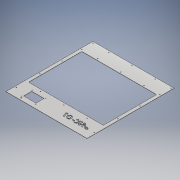
# Autodesk Inventor part: Front Cladding
Saved by Autodesk Inventor 2019 (Build 230136000, 136)
## iProperties
Created: 2018-10-13
Part Number: Front Cladding
Material: Aluminium 1050
Document SubType Name: Sheet Metal
Designer: Ax
Density: 2.7 g/cm^3
Sheet Metal Rule: Default_mm
Appearance: Anodized - Black
Mass: 471.716 g
Surface Area: 2405.62 cm^2
Volume: 174.71 cm^3
Flat Pattern Width: 51.3 cm
Flat Pattern Length: 55 cm
Flat Pattern Area: 2821.5 cm^2
Sheet Metal Width: 513.000 mm
Sheet Metal Length: 550.000 mm
Sheet Metal Area: 282150.000 mm^2
Author: Ax
Autodesk Inventor part; units mm, degrees
ref_plane "YZ Plane" through (0, 0, 0) normal (1, 0, 0) x (0, 1, 0)
ref_plane "XZ Plane" through (0, 0, 0) normal (0, 1, 0) x (-1, 0, 0)
ref_plane "XY Plane" through (0, 0, 0) normal (0, 0, 1) x (1, 0, 0)
sketch "Sketch6" plane through (0, 0, 0) normal (0, 0, -1) x (-1, 0, 0)
  line L0 (-182.0134, -208.3085) -> (-165.3558, -208.3085)
  line L1 (-165.3558, -208.3085) -> (-165.3558, -210.3085)
  line L2 (-165.3558, -210.3085) -> (-182.0134, -210.3085)
  line L3 (-182.0134, -210.3085) -> (-182.0134, -208.3085)
  line L4 (-85.6501, -195.172) -> (-83.6501, -195.172)
  line L5 (-83.6501, -195.172) -> (-83.6501, -232.9934)
  line L6 (-83.6501, -232.9934) -> (-85.6501, -232.9934)
  line L7 (-85.6501, -232.9934) -> (-85.6501, -195.172)
  line L8 (-204.8344, -216.2286) -> (-188.1555, -229.1813)
  line L9 (-188.1555, -229.1813) -> (-186.9288, -227.6017)
  line L10 (-186.9288, -227.6017) -> (-203.6076, -214.649)
  line L11 (-203.6076, -214.649) -> (-204.8344, -216.2286)
  point P0 (0, 0)
  dimension "d49" = 2
  dimension "d51" = 2
  dimension "d52" = 37.8214
  measures "d49" distance of L0.end L1.end
  measures "d51" distance of L4.start L4.end
  measures "d52" distance of L6.end L4.start
sketch "Sketch1" plane through (0, 0, 0) normal (0, 0, 1) x (1, 0, 0)
  line L0 (-256.5, -275) -> (256.5, -275)
  line L1 (256.5, -275) -> (256.5, 275)
  line L2 (256.5, 275) -> (-256.5, 275)
  line L3 (-256.5, 275) -> (-256.5, -275)
  line L4 (-256.5, -275) -> (256.5, 275) construction
  line L5 (256.5, -275) -> (-256.5, 275) construction
  line L6 (-256.5, 265) -> (256.5, 265) construction
  line L7 (-246.5, 275) -> (-246.5, -275) construction
  line L8 (246.5, 275) -> (246.5, -275) construction
  line L9 (-256.5, -165) -> (256.5, -165) construction
  line L10 (-256.5, 195) -> (256.5, 195) construction
  circle A0 centre (-246.5, 265) radius 2.1
  circle A1 centre (-146.5, 265) radius 2.1
  circle A2 centre (146.5, 265) radius 2.1
  circle A3 centre (246.5, 265) radius 2.1
  circle A4 centre (146.5, 195) radius 2.1
  circle A5 centre (246.5, 195) radius 2.1
  circle A6 centre (-246.5, 195) radius 2.1
  circle A7 centre (-146.5, 195) radius 2.1
  line L11 (-146.5, 275) -> (-146.5, -275) construction
  line L12 (0, 0) -> (0, -275) construction
  line L13 (146.5, 275) -> (146.5, -275) construction
  circle A8 centre (-246.5, 70) radius 2.1
  circle A9 centre (146.5, -165) radius 2.1
  circle A10 centre (-146.5, -165) radius 2.1
  circle A11 centre (-246.5, -70) radius 2.1
  circle A12 centre (-246.5, -220) radius 2.1
  circle A13 centre (246.5, -220) radius 2.1
  circle A14 centre (246.5, -70) radius 2.1
  circle A15 centre (246.5, 70) radius 2.1
  line L14 (-246.5, 70) -> (246.5, 70) construction
  line L15 (-246.5, -70) -> (246.5, -70) construction
  line L16 (-246.5, 0) -> (246.5, 0) construction
  line L17 (-246.5, -220) -> (246.5, -220) construction
  line L18 (0, 275) -> (0, 0) construction
  circle A16 centre (0, 265) radius 2.1
  circle A17 centre (0, 195) radius 2.1
  circle A18 centre (0, -165) radius 2.1
  line L19 (-236.5, -152) -> (236.5, -152)
  line L20 (236.5, -152) -> (236.5, 185)
  line L21 (236.5, 185) -> (-236.5, 185)
  line L22 (-236.5, 185) -> (-236.5, -152)
  dimension "d0" = 513
  dimension "d1" = 550
  dimension "d2" = 10
  dimension "d3" = 10
  dimension "d4" = 10
  dimension "d5" = 110
  dimension "d6" = 80
  dimension "d7" = 110
  dimension "d8" = 110
  dimension "d9" = 70
  dimension "d10" = 55
  dimension "d11" = 4.2
  dimension "d14" = 10
  dimension "d15" = 10
  dimension "d17" = 13
  dimension "d18" = 10
  measures "d0" distance of L1.end L2.end
  measures "d1" distance of L0.end L1.end
  measures "d2" distance of L2.end L6.start
  measures "d3" distance of L0.start L7.end
  measures "d4" distance of L0.end L8.end
  measures "d5" distance of L0.end L9.end
  measures "d6" distance of L10.end L1.end
  measures "d7" distance of L0.start L11.end
  measures "d8" distance of L13.end L0.end
  measures "d9" vertical distance of L12.start L14.start
  measures "d10" vertical distance of L0.end L17.end
  measures "d11" diameter of A7
  measures "d14" distance between parallel lines of L10 L21
  measures "d15" distance between parallel lines of L8 L20
  measures "d17" distance from line of L9 L19.end
  measures "d18" distance between parallel lines of L7 L22
extrude "Plate4" add sketch "Sketch1" along normal blind 1.5
fillet "Fillet1" radius 5 4 edges at (-236.5, 185, 0.75) (236.5, 185, 0.75) (236.5, -152, 0.75) (-236.5, -152, 0.75)
sketch "Sketch2" plane through (0, 0, 1.5) normal (0, 0, 1) x (1, 0, 0)
  line L0 (-176.5, -192) -> (-98.05, -192)
  line L1 (-98.05, -192) -> (-98.05, -243)
  line L2 (-98.05, -243) -> (-176.5, -243)
  line L3 (-176.5, -243) -> (-176.5, -192)
  line L4 (256.5, 275) -> (256.5, -275) projected
  line L5 (231.5, -152) -> (-231.5, -152) projected
  line L6 (-256.5, -275) -> (-256.5, 275) projected
  point P0 (0, 0)
  dimension "d22" = 78.45
  dimension "d23" = 51
  dimension "d25" = 40
  dimension "d28" = 80
  constraints: 8 end point, 2 parallel, 1 horizontal, 1 perpendicular
  measures "d22" distance of L0.start L0.end
  measures "d23" distance of L0.end L1.end
  measures "d25" distance between parallel lines of L0 L5
  measures "d28" distance between parallel lines of L3 L6
extrude "Cut1" cut sketch "Sketch2" against normal blind 1.5
sketch "Sketch3" plane through (0, 0, 0) normal (0, 0, -1) x (-1, 0, 0)
  circle A0 centre (173.45, -261.3) radius 3.25
  line L0 (176.5, -243) -> (98.05, -243) projected
  point P0 (0, 0)
  dimension "d29" = 6.5
  dimension "d30" = 18.3
  dimension "d31" = 3.05
  constraints: 1 centre point
  measures "d29" diameter of A0
  measures "d30" distance from line of A0.centre L0
  measures "d31" horizontal distance of L0.start A0.centre
extrude "Cut2" cut sketch "Sketch3" against normal blind 1.5
sketch "Sketch4" plane through (0, 0, 0) normal (0, 0, -1) x (-1, 0, 0)
  line L0 (93.3, -250) -> (181.25, -250) construction
  line L1 (181.25, -250) -> (181.25, -185) construction
  line L2 (181.25, -185) -> (93.3, -185) construction
  line L3 (93.3, -185) -> (93.3, -250) construction
  line L4 (93.3, -250) -> (181.25, -185) construction
  line L5 (181.25, -250) -> (93.3, -185) construction
  line L6 (98.05, -243) -> (98.05, -192) construction
  line L7 (98.05, -217.5) -> (176.5, -217.5) construction
  line L8 (176.5, -192) -> (176.5, -243) construction
  circle A0 centre (181.25, -185) radius 1.7
  circle A1 centre (181.25, -250) radius 1.7
  circle A2 centre (93.3, -250) radius 1.7
  circle A3 centre (93.3, -185) radius 1.7
  point P0 (0, 0)
  point P1 (137.275, -217.5)
  point P2 (137.275, -217.5)
  dimension "d34" = 87.95
  dimension "d35" = 65
  dimension "d36" = 3.4
  constraints: 14 end point, 6 midpoint, 4 centre point, 4 coincident, 3 equal radius, 2 parallel, 2 perpendicular, 1 horizontal
  measures "d34" distance of L0.start L0.end
  measures "d35" distance of L2.end L0.start
  measures "d36" diameter of A0
hole "Hole1" at (-181.25, -250, 0) at (-181.25, -185, 0) at (-93.3, -185, 0) at (-93.3, -250, 0) direction (0, 0, 1) diameter 3.4 end through all
sketch "Sketch5" plane through (0, 0, 0) normal (0, 0, -1) x (-1, 0, 0)
  line L0 (-179.5318, -196.7353) -> (-76.9682, -196.7353) construction
  line L1 (-76.9682, -196.7353) -> (-76.9682, -230.2647) construction
  line L2 (-76.9682, -230.2647) -> (-179.5318, -230.2647) construction
  line L3 (-179.5318, -230.2647) -> (-179.5318, -196.7353) construction
  line L4 (-128.25, -196.7353) -> (-128.25, -230.2647) construction
  line L5 (231.5, -152) -> (-231.5, -152) projected
  line L6 (-256.5, -275) -> (-256.5, 275) projected
  spline S0 degree 2 poles (-150.7053, -213.6532) (-151.7777, -217.0234) (-155.8628, -217.0234) knots 0 0 0 1 1 1
  line L7 (-155.8628, -217.0234) -> (-168.3989, -217.0234)
  line L8 (-168.3989, -217.0234) -> (-172.3564, -228.0021)
  line L9 (-172.3564, -228.0021) -> (-179.9138, -228.0021)
  line L10 (-179.9138, -228.0021) -> (-175.9564, -217.0234)
  line L11 (-175.9564, -217.0234) -> (-182.4415, -217.0234)
  spline S1 degree 2 poles (-182.4415, -217.0234) (-193.0628, -229.866) (-203.2245, -229.866) knots 0 0 0 1 1 1
  spline S2 degree 2 poles (-203.2245, -229.866) (-206.1862, -229.866) (-208.2032, -228.7681) knots 0 0 0 1 1 1
  spline S3 degree 2 poles (-208.2032, -228.7681) (-210.7564, -227.3638) (-210.7564, -224.683) knots 0 0 0 1 1 1
  spline S4 degree 2 poles (-210.7564, -224.683) (-210.7564, -222.3596) (-208.867, -220.1638) knots 0 0 0 1 1 1
  spline S5 degree 2 poles (-208.867, -220.1638) (-205.8032, -216.6404) (-199.5989, -214.9553) knots 0 0 0 1 1 1
  spline S6 degree 2 poles (-199.5989, -214.9553) (-194.7479, -213.6532) (-188.8755, -213.6532) knots 0 0 0 1 1 1
  line L12 (-188.8755, -213.6532) -> (-184.7904, -213.6532)
  line L13 (-184.7904, -213.6532) -> (-172.05, -198.3085)
  line L14 (-172.05, -198.3085) -> (-161.8117, -198.3085)
  line L15 (-161.8117, -198.3085) -> (-167.25, -213.6532)
  line L16 (-167.25, -213.6532) -> (-150.7053, -213.6532)
  spline S7 degree 2 poles (-187.6245, -217.0234) (-195.5394, -217.0234) (-198.7309, -219.2957) knots 0 0 0 1 1 1
  spline S8 degree 2 poles (-198.7309, -219.2957) (-201.3606, -221.2106) (-201.3606, -223.3553) knots 0 0 0 1 1 1
  spline S9 degree 2 poles (-201.3606, -223.3553) (-201.3606, -225.1681) (-199.4713, -225.1681) knots 0 0 0 1 1 1
  spline S10 degree 2 poles (-199.4713, -225.1681) (-196.8415, -225.1681) (-192.9351, -222.2064) knots 0 0 0 1 1 1
  spline S11 degree 2 poles (-192.9351, -222.2064) (-189.4883, -219.6532) (-187.6245, -217.0234) knots 0 0 0 1 1 1
  line L17 (-170.3904, -201.8064) -> (-179.633, -213.6532)
  line L18 (-179.633, -213.6532) -> (-174.9351, -213.6532)
  line L19 (-174.9351, -213.6532) -> (-170.3904, -201.8064)
  spline S12 degree 2 poles (-119.1989, -202.1894) (-119.1989, -204.3851) (-120.9351, -205.8404) knots 0 0 0 1 1 1
  spline S13 degree 2 poles (-120.9351, -205.8404) (-122.5692, -207.2447) (-124.7649, -207.2447) knots 0 0 0 1 1 1
  spline S14 degree 2 poles (-124.7649, -207.2447) (-126.2457, -207.2447) (-129.1819, -205.7128) (-129.9734, -204.4872) knots 0 0 0 1 2 2 2
  line L20 (-129.9734, -204.4872) -> (-137.0968, -211.9681)
  line L21 (-137.0968, -211.9681) -> (-133.7777, -224.6319)
  line L22 (-133.7777, -224.6319) -> (-122.7479, -224.6319)
  spline S15 degree 2 poles (-122.7479, -224.6319) (-123.0287, -226.2915) (-124.7649, -227.2106) knots 0 0 0 1 1 1
  spline S16 degree 2 poles (-124.7649, -227.2106) (-126.2202, -228.0021) (-128.0585, -228.0021) knots 0 0 0 1 1 1
  line L23 (-128.0585, -228.0021) -> (-136.3564, -228.0021)
  spline S17 degree 2 poles (-136.3564, -228.0021) (-138.4245, -228.0021) (-139.9053, -226.7511) knots 0 0 0 1 1 1
  spline S18 degree 2 poles (-139.9053, -226.7511) (-141.3096, -225.5511) (-141.8968, -223.5596) knots 0 0 0 1 1 1
  line L24 (-141.8968, -223.5596) -> (-143.3266, -218.683)
  line L25 (-143.3266, -218.683) -> (-150.067, -225.7043)
  spline S19 degree 2 poles (-150.067, -225.7043) (-152.7989, -228.5638) (-155.9394, -228.5638) knots 0 0 0 1 1 1
  spline S20 degree 2 poles (-155.9394, -228.5638) (-158.1606, -228.5638) (-159.8202, -227.1596) knots 0 0 0 1 1 1
  spline S21 degree 2 poles (-159.8202, -227.1596) (-161.5564, -225.7043) (-161.5564, -223.483) knots 0 0 0 1 1 1
  spline S22 degree 2 poles (-161.5564, -223.483) (-161.5564, -221.3894) (-158.2628, -218.4277) (-155.9394, -218.4277) knots 0 0 0 1 2 2 2
  spline S23 degree 2 poles (-155.9394, -218.4277) (-152.4415, -218.4277) (-150.884, -221.3383) knots 0 0 0 1 1 1
  line L26 (-150.884, -221.3383) -> (-144.45, -214.5979)
  line L27 (-144.45, -214.5979) -> (-147.0287, -203.6191)
  line L28 (-147.0287, -203.6191) -> (-157.5223, -203.6191)
  line L29 (-157.5223, -203.6191) -> (-154.3309, -198.3085)
  line L30 (-154.3309, -198.3085) -> (-145.4713, -198.3085)
  spline S24 degree 2 poles (-145.4713, -198.3085) (-139.9819, -198.3085) (-139.0372, -202.8787) knots 0 0 0 1 1 1
  line L31 (-139.0372, -202.8787) -> (-138.016, -207.8574)
  line L32 (-138.016, -207.8574) -> (-131.7096, -201.2702)
  spline S25 degree 2 poles (-131.7096, -201.2702) (-129.4372, -198.8957) (-128.7223, -198.3851) knots 0 0 0 1 1 1
  spline S26 degree 2 poles (-128.7223, -198.3851) (-127.0117, -197.134) (-124.816, -197.134) knots 0 0 0 1 1 1
  spline S27 degree 2 poles (-124.816, -197.134) (-122.5947, -197.134) (-120.9351, -198.5383) knots 0 0 0 1 1 1
  spline S28 degree 2 poles (-120.9351, -198.5383) (-119.1989, -199.9936) (-119.1989, -202.1894) knots 0 0 0 1 1 1
  line L33 (-105.667, -215.7213) -> (-107.5309, -221.083)
  line L34 (-107.5309, -221.083) -> (-121.7521, -221.083)
  line L35 (-121.7521, -221.083) -> (-119.8883, -215.7213)
  line L36 (-119.8883, -215.7213) -> (-105.667, -215.7213)
  spline S29 degree 2 poles (-69.8202, -211.3809) (-69.8202, -218.683) (-74.084, -223.4319) knots 0 0 0 1 1 1
  spline S30 degree 2 poles (-74.084, -223.4319) (-78.5266, -228.334) (-85.7521, -228.334) knots 0 0 0 1 1 1
  spline S31 degree 2 poles (-85.7521, -228.334) (-91.5734, -228.334) (-98.6457, -221.2362) (-98.6457, -215.3894) knots 0 0 0 1 2 2 2
  spline S32 degree 2 poles (-98.6457, -215.3894) (-98.6457, -208.1128) (-94.3309, -203.3128) knots 0 0 0 1 1 1
  spline S33 degree 2 poles (-94.3309, -203.3128) (-89.8883, -198.3596) (-82.6883, -198.3596) knots 0 0 0 1 1 1
  spline S34 degree 2 poles (-82.6883, -198.3596) (-76.8415, -198.3596) (-69.8202, -205.534) (-69.8202, -211.3809) knots 0 0 0 1 2 2 2
  spline S35 degree 2 poles (-78.8585, -208.9553) (-78.8585, -202.6745) (-82.5351, -202.6745) knots 0 0 0 1 1 1
  spline S36 degree 2 poles (-82.5351, -202.6745) (-86.1096, -202.6745) (-88.2032, -208.8277) knots 0 0 0 1 1 1
  spline S37 degree 2 poles (-88.2032, -208.8277) (-89.7862, -213.4489) (-89.7862, -218.0191) knots 0 0 0 1 1 1
  spline S38 degree 2 poles (-89.7862, -218.0191) (-89.7862, -224.2489) (-86.084, -224.2489) knots 0 0 0 1 1 1
  spline S39 degree 2 poles (-86.084, -224.2489) (-82.4585, -224.2489) (-80.3904, -218.1213) knots 0 0 0 1 1 1
  spline S40 degree 2 poles (-80.3904, -218.1213) (-78.8585, -213.5511) (-78.8585, -208.9553) knots 0 0 0 1 1 1
  line L37 (-50.2883, -204.0787) -> (-57.8968, -228.0021)
  line L38 (-57.8968, -228.0021) -> (-65.5053, -228.0021)
  line L39 (-65.5053, -228.0021) -> (-57.9223, -203.6702)
  line L40 (-57.9223, -203.6702) -> (-63.8457, -203.6702)
  line L41 (-63.8457, -203.6702) -> (-61.1904, -198.3085)
  line L42 (-61.1904, -198.3085) -> (-53.3777, -198.3085)
  spline S41 degree 2 poles (-53.3777, -198.3085) (-51.8202, -198.3085) (-50.8755, -199.2277) knots 0 0 0 1 1 1
  spline S42 degree 2 poles (-50.8755, -199.2277) (-49.8543, -200.1979) (-49.8543, -201.8319) knots 0 0 0 1 1 1
  spline S43 degree 2 poles (-49.8543, -201.8319) (-49.8543, -202.8787) (-50.2883, -204.0787) knots 0 0 0 1 1 1
  point P0 (0, 0)
  point P1 (-128.25, -213.5)
  dimension "d44" = 61.5
  dimension "d46" = 128.25
  constraints: 3 midpoint, 2 end point, 2 other
  measures "d44" distance from line of point (-128.25, -213.5) L5
  measures "d46" distance from line of point (-128.25, -213.5) L6
extrude "Extrusion1" cut sketch "Sketch5" against normal blind 10
sheet face with bend "Face5" sketch "Sketch6" thickness 1.5 toward (0, 0, 1) bend radius 0.8
bend "Bend1"
equation "\"d26\" = Thickness"
equation "\"d32\" = Thickness"
equation "\"d42\" = Thickness"
equation "\"d51\" = d49"
equation "\"d21\" = Thickness"
equation "\"d53\" = BendRadius"
equation "\"d54\" = BendReliefWidth"
equation "\"d56\" = MinimumRemnant"
equation "\"d55\" = BendReliefDepth"
equation "\"d57\" = TransitionRadius"
equation "\"CornerReliefSize\" = 4 * Thickness"
equation "\"TransitionRadius\" = BendRadius"
equation "\"JacobiRadiusSize\" = BendRadius"
equation "\"d12\" = BendRadius"
equation "\"d13\" = BendRadius"
equation "\"d16\" = BendRadius"
equation "\"d19\" = BendRadius"
equation "\"Thickness\" = 1.5"
equation "\"BendRadius\" = 0.8"
equation "\"BendReliefWidth\" = 0.2"
equation "\"MinimumRemnant\" = 0.2"
equation "\"BendReliefDepth\" = 0.2"
body "Solid4"
